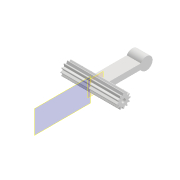
# Autodesk Inventor part: 40_Light-sheet_Z_mechanism_levelarm
Saved by Autodesk Inventor 2022 (Build 260153000, 153)
## iProperties
Created: 2021-05-14
Part Number: 40_Light-sheet_Z_mechanism_levelarm
Material: Generic
Document SubType Name: Modeling
Designer: diederichbenedict
Density: 1 g/cm^3
Appearance: Default
Author: diederichbenedict
Autodesk Inventor part; units mm, degrees
ref_plane "YZ Plane" through (0, 0, 0) normal (1, 0, 0) x (0, 1, 0)
ref_plane "XZ Plane" through (0, 0, 0) normal (0, 1, 0) x (-1, 0, 0)
ref_plane "XY Plane" through (0, 0, 0) normal (0, 0, 1) x (1, 0, 0)
ref_plane "Work Plane1" through (-11.1225, -8.6007, 24.2188) normal (-1, 0, 0) x (0, 0, 1)
sketch "Sketch1" plane through (-11.1225, -8.6007, 24.2188) normal (-1, 0, 0) x (0, 0, 1)
  line L0 (-16.0994, 9.698) -> (-17.9787, 9.014) projected
  line L1 (-17.9787, 9.014) -> (-17.9787, 8.614) projected
  line L2 (-17.9787, 8.614) -> (-16.0994, 7.9299) projected
  line L3 (-16.0994, 9.698) -> (-16.0994, 7.9299) projected
  circle A0 centre (-21.4394, 8.8293) radius 3.4607
  line L4 (-17.9787, 8.8293) -> (-16.3492, 8.8293)
  line L5 (-16.3492, 8.8293) -> (-16.3492, 8.9793)
  line L6 (-16.3492, 8.9793) -> (-18.0667, 9.6044)
  line L7 (-16.3492, 8.8293) -> (-16.3492, 8.6293)
  line L8 (-16.3492, 8.8293) -> (-16.1492, 8.8293) construction
  line L9 (-16.3492, 8.6293) -> (-18.0797, 7.9994)
  point P0 (-24.2188, 8.6007)
  dimension "d0" = 0.15
  dimension "d1" = 110
  dimension "d2" = 0.2
  dimension "d3" = 90
  dimension "a1" = 110
  constraints: 12 end point, 3 point on circle, 2 horizontal, 2 perpendicular, 1 centre point, 1 point on line, 1 tangent, 1 vertical
  measures "d0" distance of L4.end L5.end
  measures "d1" angle of L5 L6
  measures "d2" distance of L4.end L7.end
  measures "d3" angle of L7 L8
  measures "a1" angle of L7 L9
extrude "Extrusion1" add sketch "Sketch1" along normal mid plane 40 contours L6 L5 L4 L1 L0 | L0 L1 A0 L6 | A0 | L9 A0 L1 L2 | L2 L1 L4 L7 L9
fillet "Fillet1" radius 0.3 4 edges at (-11.1225, 1.0037, 6.1521) (-11.1225, 0.3786, 7.8696) (-11.1225, 0.0286, 7.8696) (-11.1225, -0.6013, 6.1391)
pattern_circular "Circular Pattern2" count 12 over 360 about axis through (-11.1225, 0.2286, 2.7794) along (-1, 0, 0) of "Extrusion1", "Fillet1"
ref_plane "Work Plane2" through (-11.1225, -8.6007, 24.2188) normal (1, 0, 0) x (0, 0, -1)
sketch "Sketch2" plane through (8.8775, -8.6007, 24.2188) normal (1, 0, 0) x (0, 0, -1)
  arc A0 (17.9175, 9.5501) -> (18.0845, 9.7005) centre (17.8149, 9.832) ccw projected
  line L0 (17.9175, 9.5501) -> (16.6429, 9.0862) projected
  arc A1 (16.6429, 9.0862) -> (16.6429, 8.5223) centre (16.7455, 8.8043) ccw projected
  line L1 (16.6429, 8.5223) -> (17.9334, 8.0527) projected
  arc A2 (18.0984, 7.9064) -> (17.9334, 8.0527) centre (17.8308, 7.7708) ccw projected
  arc A3 (18.0289, 7.6925) -> (18.0984, 7.9064) centre (17.7991, 7.8854) ccw projected
  line L2 (18.0289, 7.6925) -> (17.1571, 6.6535) projected
  arc A4 (17.1571, 6.6535) -> (17.439, 6.1652) centre (17.3869, 6.4607) ccw projected
  line L3 (17.439, 6.1652) -> (18.7914, 6.4037) projected
  arc A5 (19.0075, 6.3595) -> (18.7914, 6.4037) centre (18.8435, 6.1082) ccw projected
  arc A6 (19.0542, 6.1396) -> (19.0075, 6.3595) centre (18.7588, 6.1917) ccw projected
  line L4 (19.0542, 6.1396) -> (18.8187, 4.8038) projected
  arc A7 (18.8187, 4.8038) -> (19.307, 4.5219) centre (19.1141, 4.7517) ccw projected
  line L5 (19.307, 4.5219) -> (20.359, 5.4046) projected
  arc A8 (20.5682, 5.4744) -> (20.359, 5.4046) centre (20.5518, 5.1748) ccw projected
  arc A9 (20.7186, 5.3073) -> (20.5682, 5.4744) centre (20.4367, 5.2047) ccw projected
  line L6 (20.7186, 5.3073) -> (21.1825, 4.0328) projected
  arc A10 (21.1825, 4.0328) -> (21.7463, 4.0328) centre (21.4644, 4.1354) ccw projected
  line L7 (21.7463, 4.0328) -> (22.216, 5.3232) projected
  arc A11 (22.3623, 5.4882) -> (22.216, 5.3232) centre (22.4979, 5.2206) ccw projected
  arc A12 (22.5762, 5.4188) -> (22.3623, 5.4882) centre (22.3833, 5.1889) ccw projected
  line L8 (22.5762, 5.4188) -> (23.6152, 4.5469) projected
  arc A13 (23.6152, 4.5469) -> (24.1035, 4.8288) centre (23.808, 4.7767) ccw projected
  line L9 (24.1035, 4.8288) -> (23.865, 6.1812) projected
  arc A14 (23.9092, 6.3973) -> (23.865, 6.1812) centre (24.1604, 6.2333) ccw projected
  arc A15 (24.1291, 6.4441) -> (23.9092, 6.3973) centre (24.077, 6.1486) ccw projected
  line L10 (24.1291, 6.4441) -> (25.4649, 6.2085) projected
  arc A16 (25.4649, 6.2085) -> (25.7468, 6.6968) centre (25.5169, 6.504) ccw projected
  line L11 (25.7468, 6.6968) -> (24.864, 7.7488) projected
  arc A17 (24.7943, 7.958) -> (24.864, 7.7488) centre (25.0939, 7.9416) ccw projected
  arc A18 (24.9614, 8.1085) -> (24.7943, 7.958) centre (25.064, 7.8265) ccw projected
  line L12 (24.9614, 8.1085) -> (26.2359, 8.5723) projected
  arc A19 (26.2359, 8.5723) -> (26.2359, 9.1362) centre (26.1333, 8.8543) ccw projected
  line L13 (26.2359, 9.1362) -> (24.9455, 9.6058) projected
  arc A20 (24.7805, 9.7522) -> (24.9455, 9.6058) centre (25.0481, 9.8878) ccw projected
  arc A21 (24.8499, 9.966) -> (24.7805, 9.7522) centre (25.0797, 9.7732) ccw projected
  line L14 (24.8499, 9.966) -> (25.7218, 11.005) projected
  arc A22 (25.7218, 11.005) -> (25.4399, 11.4933) centre (25.4919, 11.1978) ccw projected
  line L15 (25.4399, 11.4933) -> (24.0875, 11.2548) projected
  arc A23 (23.8714, 11.299) -> (24.0875, 11.2548) centre (24.0354, 11.5503) ccw projected
  arc A24 (23.8246, 11.5189) -> (23.8714, 11.299) centre (24.1201, 11.4669) ccw projected
  line L16 (23.8246, 11.5189) -> (24.0602, 12.8547) projected
  arc A25 (24.0602, 12.8547) -> (23.5719, 13.1366) centre (23.7647, 12.9068) ccw projected
  line L17 (23.5719, 13.1366) -> (22.5199, 12.2539) projected
  arc A26 (22.3107, 12.1841) -> (22.5199, 12.2539) centre (22.3271, 12.4837) ccw projected
  arc A27 (22.1602, 12.3512) -> (22.3107, 12.1841) centre (22.4421, 12.4538) ccw projected
  line L18 (22.1602, 12.3512) -> (21.6963, 13.6257) projected
  arc A28 (21.6963, 13.6257) -> (21.1325, 13.6257) centre (21.4144, 13.5231) ccw projected
  line L19 (21.1325, 13.6257) -> (20.6628, 12.3353) projected
  arc A29 (20.5165, 12.1703) -> (20.6628, 12.3353) centre (20.3809, 12.4379) ccw projected
  arc A30 (20.3027, 12.2397) -> (20.5165, 12.1703) centre (20.4955, 12.4696) ccw projected
  line L20 (20.3027, 12.2397) -> (19.2637, 13.1116) projected
  arc A31 (19.2637, 13.1116) -> (18.7754, 12.8297) centre (19.0708, 12.8818) ccw projected
  line L21 (18.7754, 12.8297) -> (19.0139, 11.4773) projected
  arc A32 (18.9696, 11.2612) -> (19.0139, 11.4773) centre (18.7184, 11.4252) ccw projected
  arc A33 (18.7497, 11.2145) -> (18.9696, 11.2612) centre (18.8018, 11.5099) ccw projected
  line L22 (18.7497, 11.2145) -> (17.414, 11.45) projected
  arc A34 (17.414, 11.45) -> (17.1321, 10.9617) centre (17.3619, 11.1545) ccw projected
  line L23 (17.1321, 10.9617) -> (18.0148, 9.9097) projected
  arc A35 (18.0845, 9.7005) -> (18.0148, 9.9097) centre (17.785, 9.7169) ccw projected
  circle A36 centre (21.4144, 8.8043) radius 1.4
  point P0 (24.2188, 8.6007)
  dimension "d14" = 2.8
  constraints: 1 centre point
  measures "d14" diameter of A36
extrude "Extrusion2" cut sketch "Sketch2" against normal through all contours A36
sketch "Sketch4" plane through (-11.1225, -8.6007, 24.2188) normal (1, 0, 0) x (0, 0, -1)
  circle A0 centre (21.4144, 8.8043) radius 1.4 projected
  line L0 (51.213, 10.8043) -> (24.8312, 10.8043)
  line L1 (24.8312, 10.8043) -> (24.8312, 6.8043)
  line L2 (24.8312, 6.8043) -> (51.213, 6.8043)
  line L3 (51.213, 6.8043) -> (51.213, 10.8043)
  line L4 (51.213, 10.8043) -> (24.8312, 6.8043) construction
  line L5 (24.8312, 10.8043) -> (51.213, 6.8043) construction
  circle A1 centre (52.5846, 8.8043) radius 4.4101
  point P0 (24.2188, 8.6007)
  point P1 (38.0221, 8.8043)
  dimension "d20" = 4
  constraints: 12 end point, 2 midpoint, 2 parallel, 1 centre point, 1 horizontal, 1 perpendicular
  measures "d20" distance of L1.end L0.end
extrude "Extrusion3" add sketch "Sketch4" along normal mid plane 10 contours L3 L2 A1 L0 | L0 A1 L2 L3 | A1 L2 L1 L0
equation "\"d1\" = a1"
body "Solid1"
